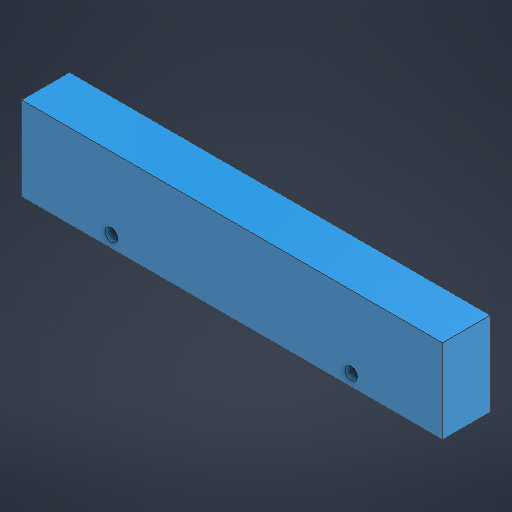
# Autodesk Inventor part: Coupler
Saved by Autodesk Inventor 2026.2 (Build 302298010, 298A)
## iProperties
Created: 2026-06-11
Part Number: Coupler
Material: Generic
Document SubType Name: Modeling
Designer: sonata
Density: 1 g/cm^3
Appearance: Default
Author: sonata
Autodesk Inventor part; units mm, degrees
ref_plane "YZ Plane" through (0, 0, 0) normal (1, 0, 0) x (0, 1, 0)
ref_plane "XZ Plane" through (0, 0, 0) normal (0, 1, 0) x (-1, 0, 0)
ref_plane "XY Plane" through (0, 0, 0) normal (0, 0, 1) x (1, 0, 0)
sketch "Sketch1" plane through (0, 0, 0) normal (0, 0, 1) x (1, 0, 0)
  line L0 (0, 0) -> (89.154, 0)
  line L1 (89.154, 0) -> (89.154, 17.78)
  line L2 (89.154, 17.78) -> (0, 17.78)
  line L3 (0, 17.78) -> (0, 0)
  dimension "d0" = 89.154
  dimension "d1" = 17.78
  constraints: 8 end point, 2 parallel, 1 horizontal, 1 perpendicular
  measures "d0" distance of L1.end L2.end
  measures "d1" distance of L0.end L1.end
extrude "Extrusion1" add sketch "Sketch1" along normal blind 10.16
sketch "Sketch2" plane through (0, 0, 10.16) normal (0, 0, 1) x (1, 0, 0)
  line L0 (0, 17.78) -> (0, 0) projected
  line L1 (0, 0) -> (89.154, 0) projected
  point P0 (19.05, 2.54)
  point P1 (69.85, 2.54)
  point P2 (0, 8.89)
  dimension "d4" = 19.05
  dimension "d5" = 50.8
  dimension "d6" = 2.54
  constraints: 1 horizontal alignment, 1 midpoint
  measures "d4" horizontal distance of point (19.05, 2.54) point (0, 8.89)
  measures "d5" distance of point (69.85, 2.54) point (19.05, 2.54)
  measures "d6" distance from line of point (19.05, 2.54) L1
hole "Hole1" at (19.05, 2.54, 10.16) at (69.85, 2.54, 10.16) direction (0, 0, -1) diameter 2.667 end through all
body "Solid1"
